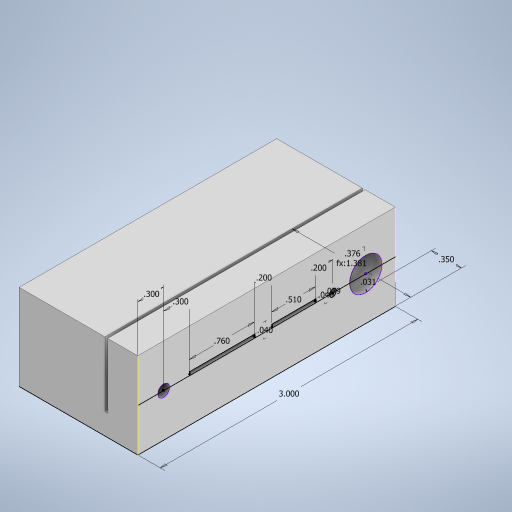
# Autodesk Inventor part: Cutting Jig
Saved by Autodesk Inventor 2023 (Build 270158000, 158)
## iProperties
Created: 2023-04-01
Part Number: Cutting Jig
Material: Generic
Document SubType Name: Modeling
Designer: tommy
Density: 1 g/cm^3
Appearance: Default
Author: tommy
Autodesk Inventor part; units mm, degrees
ref_plane "YZ Plane" through (0, 0, 0) normal (1, 0, 0) x (0, 1, 0)
ref_plane "XZ Plane" through (0, 0, 0) normal (0, 1, 0) x (-1, 0, 0)
ref_plane "XY Plane" through (0, 0, 0) normal (0, 0, 1) x (1, 0, 0)
sketch "Sketch1" plane through (0, 0, 0) normal (0, 1, 0) x (-1, 0, 0)
  line L0 (0, 0) -> (0, -76.2)
  line L1 (0, -76.2) -> (35.09, -76.2)
  line L2 (35.09, -76.2) -> (35.09, 0)
  line L3 (35.09, 0) -> (0, 0)
  line L4 (8.89, 0) -> (8.89, -76.2)
  line L5 (9.69, 0) -> (9.69, -76.2)
  dimension "d1" = 76.2
  dimension "d2" = 35.09
  dimension "d3" = 8.89
  dimension "d4" = 0.8
  constraints: 12 end point, 5 perpendicular, 4 point on line, 1 vertical
  measures "d1" distance of L0.start L0.end
  measures "d2" distance of L0.end L1.end
  measures "d3" distance between parallel lines of L0 L4
  measures "d4" distance between parallel lines of L4 L5
extrude "Extrusion1" add sketch "Sketch1" along normal blind 6.35
extrude "Extrusion2" add sketch "Sketch1" along normal blind 25.4 contours L3 L4 L1 L0
extrude "Extrusion3" add sketch "Sketch1" along normal blind 25.4 contours L3 L2 L1 L5
sketch "Sketch2" plane through (0, 0, 0) normal (1, 0, 0) x (0, 0, -1)
  line L0 (0, 0) -> (0, 25.4) projected
  line L1 (0, 12.7) -> (76.2, 12.7)
  line L2 (76.2, 6.35) -> (76.2, 25.4) projected
  circle A0 centre (7.62, 12.7) radius 1.716
  line L3 (15.24, 12.7) -> (34.544, 12.7)
  line L4 (34.544, 12.7) -> (34.544, 13.716)
  line L5 (34.544, 13.716) -> (15.24, 13.716)
  line L6 (15.24, 13.716) -> (15.24, 12.7)
  line L7 (39.624, 12.7) -> (52.578, 12.7)
  line L8 (52.578, 12.7) -> (52.578, 13.716)
  line L9 (52.578, 13.716) -> (39.624, 13.716)
  line L10 (39.624, 13.716) -> (39.624, 12.7)
  circle A1 centre (57.658, 12.7) radius 1.0033
  circle A2 centre (67.4281, 12.7) radius 4.7752
  point P0 (15.24, 13.208)
  point P1 (39.624, 13.208)
  point P2 (34.544, 13.208)
  point P3 (52.578, 13.208)
  dimension "d13" = 19.304
  dimension "d14" = 1.016
  dimension "d15" = 12.954
  dimension "d16" = 1.016
  dimension "d19" = 2.0066
  dimension "d22" = 7.62
  dimension "d23" = 7.62
  dimension "d24" = 5.08
  dimension "d25" = 5.08
  dimension "d26" = 9.5504
  constraints: 18 end point, 6 point on line, 5 midpoint, 4 parallel, 3 centre point, 3 horizontal, 2 perpendicular
  measures "d13" distance of L5.end L4.end
  measures "d14" distance of L4.end L3.end
  measures "d15" distance of L9.end L8.end
  measures "d16" distance of L8.end L7.end
  measures "d19" diameter of A1
  measures "d22" distance from line of L0 A0.centre
  measures "d23" horizontal distance of A0.centre point (15.24, 13.208)
  measures "d24" distance of point (39.624, 13.208) point (34.544, 13.208)
  measures "d25" horizontal distance of point (52.578, 13.208) A1.centre
  measures "d26" diameter of A2
extrude "Extrusion4" cut sketch "Sketch2" against normal blind 28.486 contours A0 L1 | L1 A0
extrude "Extrusion5" cut sketch "Sketch2" against normal blind 27.978 contours L10 L9 L8 L1 | L6 L5 L4 L1
extrude "Extrusion6" cut sketch "Sketch2" against normal blind 18.58 contours A1 L1 | L1 A1
extrude "Extrusion7" cut sketch "Sketch2" against normal blind 11.2394 contours A2 L1 | L1 A2
body "Solid1"
